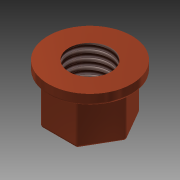
# Autodesk Inventor part: 刀轴端盖螺帽
Saved by Autodesk Inventor 2015 (Build 190159000, 159)
## iProperties
Created: 2017-05-17
Part Number: 刀轴端盖螺帽
Material: 常规
Document SubType Name: Modeling
Designer: Administrator
Density: 1 g/cm^3
Appearance: 铜 - 缎光
Author: Administrator
Autodesk Inventor part; units mm, degrees
ref_plane "YZ Plane" through (0, 0, 0) normal (1, 0, 0) x (0, 1, 0)
ref_plane "XZ Plane" through (0, 0, 0) normal (0, 1, 0) x (-1, 0, 0)
ref_plane "XY Plane" through (0, 0, 0) normal (0, 0, 1) x (1, 0, 0)
sketch "草图1" plane through (0, 0, 0) normal (0, 0, 1) x (1, 0, 0)
  circle A0 centre (0, 0) radius 2
  line L0 (1.7321, -3) -> (-1.7321, -3)
  line L1 (-1.7321, -3) -> (-3.4641, 0)
  line L2 (-3.4641, 0) -> (-1.7321, 3)
  line L3 (-1.7321, 3) -> (1.7321, 3)
  line L4 (1.7321, 3) -> (3.4641, 0)
  line L5 (3.4641, 0) -> (1.7321, -3)
  line L6 (0, 0) -> (0, 1.0765)
  point P0 (0, 3)
  dimension "d0" = 4
  dimension "d1" = 1.0765
  dimension "d2" = 6
  constraints: 14 end point, 2 coincident, 1 centre point, 1 midpoint, 1 point on line, 1 vertical, 13 other
  measures "d0" diameter of A0
  measures "d1" distance of L6.start L6.end
  measures "d2" distance between parallel lines of L0 L3
extrude "拉伸1" add sketch "草图1" along normal blind 4
sketch "草图2" plane through (0, 0, 4) normal (0, 0, 1) x (1, 0, 0)
  circle A0 centre (0, 0) radius 4
  circle A1 centre (0, 0) radius 2
  dimension "d5" = 8
  dimension "d6" = 4
  constraints: 2 centre point, 2 coincident
  measures "d5" diameter of A0
  measures "d6" diameter of A1
extrude "拉伸2" add sketch "草图2" along normal blind 1
thread "螺纹1" size "M4x0.7" class "6H" standard "ANSI Metric M Profile" full length
fillet "圆角1" radius 0.25 13 edges at (-4, 0, 4) (1.7321, 3, 2) (2.5981, 1.5, 0) (0, 3, 0) (-2.5981, 1.5, 0) (-2.5981, -1.5, 0) (0, -3, 0) (2.5981, -1.5, 0) (1.7321, -3, 2) (3.4641, 0, 2) (-1.7321, -3, 2) (-3.4641, 0, 2) (-1.7321, 3, 2)
chamfer "倒角1" distance 0.25 angle 45 1 edges at (-2, 0, 0)
